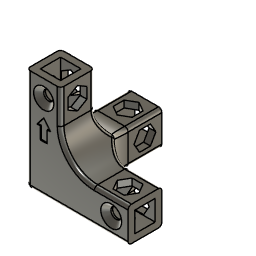
Corner Piece - Cube v1 (Autodesk Fusion 360 design; units mm, degrees)
Autodesk Fusion 360 part; units mm, degrees
sketch "Sketch5" plane through (0, 0, 0) normal (0, 0, 1) x (1, 0, 0)
  line L0 (0, 0) -> (10, 0)
  line L1 (10, 0) -> (10, 10)
  line L2 (0, 10) -> (0, 0)
  line L3 (10, 10) -> (10, 20)
  line L4 (10, 20) -> (0, 20)
  line L5 (0, 20) -> (0, 10)
  line L6 (10, 0) -> (20, 0)
  line L7 (20, 0) -> (20, 10)
  line L8 (20, 10) -> (10, 10)
  line L9 (10, 10) -> (10, 0)
  line L10 (10, 10) -> (0, 10)
  dimension "d18" = 10
  constraint horizontal L0
  constraint vertical L1
  constraint vertical L2
  constraint coincident L0.start L2.end
  constraint equal L0 L2
  constraint vertical L3
  constraint horizontal L4
  constraint vertical L5
  constraint equal L2 L5
  constraint horizontal L6
  constraint vertical L7
  constraint horizontal L8
  constraint vertical L9
  constraint perpendicular L2 L10
  constraint equal L0 L6
  constraint equal L7 L8
  constraint equal L3 L4
  constraint equal L3 L10
  measures "d18" distance of L0.start L0.end
extrude "Extrude8" add sketch "Sketch5" along normal blind 20 contours L0 L1 L2 L9 L10
extrude "Extrude9" add sketch "Sketch5" along normal blind 10 contours L1 L6 L7 L8 L9 | L3 L4 L5 L10
sketch "Sketch6" plane through (20, 0, 0) normal (1, 0, 0) x (0, 1, 0)
  line L0 (0, 0) -> (10, 0)
  line L1 (10, 0) -> (10, 10)
  line L2 (10, 10) -> (0, 10)
  line L3 (0, 10) -> (0, 0)
  line L4 (0, 10) -> (2, 10) construction
  line L5 (2, 10) -> (2, 8) construction
  line L6 (10, 0) -> (8, 0) construction
  line L7 (8, 0) -> (8, 2) construction
  line L8 (2, 8) -> (8, 8)
  line L9 (8, 8) -> (8, 2)
  line L10 (8, 2) -> (2, 2)
  line L11 (2, 2) -> (2, 8)
  dimension "CornerPeg" = 2
  dimension "d24" = 2
  dimension "d25" = 2
  dimension "d26" = 2
  constraint coincident L2.end L3.start
  constraint perpendicular L3 L4
  constraint perpendicular L4 L5
  constraint coincident L0.end L1.start
  constraint coincident L0 L6.end
  constraint perpendicular L6 L7
  constraint horizontal L8
  constraint vertical L9
  constraint horizontal L10
  constraint vertical L11
  measures "CornerPeg" distance of L2.end L4.end
  measures "d24" distance of L4.end L5.end
  measures "d25" distance of L0.end L6.end
  measures "d26" distance of L6.end L7.end
sketch "Sketch7" plane through (0, 20, 0) normal (0, 1, 0) x (-1, 0, 0)
  line L0 (-10, 0) -> (0, 0)
  line L1 (0, 0) -> (0, 10)
  line L2 (0, 10) -> (-10, 10)
  line L3 (-10, 10) -> (-10, 0)
  line L4 (0, 0) -> (-2, 0) construction
  line L5 (-2, 0) -> (-2, 2) construction
  line L6 (-10, 10) -> (-8, 10) construction
  line L7 (-8, 10) -> (-8, 8) construction
  line L8 (-8, 8) -> (-2, 8)
  line L9 (-2, 8) -> (-2, 2)
  line L10 (-2, 2) -> (-8, 2)
  line L11 (-8, 2) -> (-8, 8)
  dimension "d27" = 2
  dimension "d28" = 2
  dimension "d29" = 2
  dimension "d30" = 2
  constraint coincident L0.end L1.start
  constraint perpendicular L1 L4
  constraint perpendicular L4 L5
  constraint coincident L2.end L3.start
  constraint perpendicular L3 L6
  constraint perpendicular L6 L7
  constraint horizontal L8
  constraint vertical L9
  constraint horizontal L10
  constraint vertical L11
  measures "d27" distance of L0.end L4.end
  measures "d28" distance of L4.end L5.end
  measures "d29" distance of L2.end L6.end
  measures "d30" distance of L6.end L7.end
sketch "Sketch8" plane through (0, 0, 20) normal (0, 0, 1) x (-1, 0, 0)
  line L0 (-10, -10) -> (0, -10)
  line L1 (0, -10) -> (0, 0)
  line L2 (0, 0) -> (-10, 0)
  line L3 (-10, 0) -> (-10, -10)
  line L4 (0, -10) -> (-2, -10) construction
  line L5 (-2, -10) -> (-2, -8) construction
  line L6 (-10, 0) -> (-8, 0) construction
  line L7 (-8, 0) -> (-8, -2) construction
  line L8 (-2, -8) -> (-8, -8)
  line L9 (-8, -8) -> (-8, -2)
  line L10 (-8, -2) -> (-2, -2)
  line L11 (-2, -2) -> (-2, -8)
  dimension "d31" = 2
  dimension "d32" = 2
  dimension "d33" = 2
  dimension "d34" = 2
  constraint coincident L0.end L1.start
  constraint perpendicular L1 L4
  constraint perpendicular L0 L5
  constraint coincident L2.end L3.start
  constraint perpendicular L3 L6
  constraint perpendicular L2 L7
  constraint horizontal L8
  constraint vertical L9
  constraint horizontal L10
  constraint vertical L11
  measures "d31" distance of L0.end L4.end
  measures "d32" distance of L4.end L5.end
  measures "d33" distance of L2.end L6.end
  measures "d34" distance of L6.end L7.end
extrude "Extrude10" cut sketch "Sketch8" against normal blind 10 contours L8 L9 L10 L11
extrude "Extrude11" cut sketch "Sketch6" against normal blind 10 contours L8 L9 L10 L11
extrude "Extrude12" cut sketch "Sketch7" against normal blind 10 draft 1 contours L8 L9 L10 L11
extrude "Extrude13" add 1 faces at (20, 4, 9.3333) along direction (1, 0, 0) blind 10
extrude "Extrude14" add 1 faces at (6, 0.6667, 20) along direction (0, 0, 1) blind 10
extrude "Extrude15" add 1 faces at (4, 20, 9.3333) along direction (0, 1, 0) blind 10
fillet "Fillet1" radius 10 1 edges at (10, 10, 5)
fillet "Fillet2" radius 10 1 edges at (10, 5, 10)
fillet "Fillet3" radius 10 1 edges at (10, 10, 10)
sketch "Sketch9" plane through (0, 0, 10) normal (0, 0, 1) x (-1, 0, 0)
  line L0 (-20, -10) -> (-20, 0)
  line L1 (-20, 0) -> (-30, 0)
  line L2 (-30, 0) -> (-30, -10)
  line L3 (-30, -10) -> (-20, -10)
  line L4 (-30, -5) -> (-20, -5) construction
  circle A0 centre (-25, -5) radius 1.5
  dimension "d53" = 3
  constraint midpoint L2 L4.start
  constraint perpendicular L0 L4
  constraint midpoint L4 A0.centre
  constraint midpoint L0 L4.end
  measures "d53" diameter of A0
sketch "Sketch10" plane through (0, 0, 10) normal (0, 0, 1) x (-1, 0, 0)
  line L0 (-10, -20) -> (-10, -30)
  line L1 (-10, -30) -> (0, -30)
  line L2 (0, -30) -> (0, -20)
  line L3 (-5, -30) -> (-5, -20) construction
  circle A0 centre (-5, -25) radius 1.5
  line L4 (0, -20) -> (-10, -20)
  dimension "d54" = 3
  constraint midpoint L1 L3.start
  constraint perpendicular L1 L3
  constraint midpoint L3 A0.centre
  constraint midpoint L3.end L4
  measures "d54" diameter of A0
sketch "Sketch11" plane through (0, 10, 0) normal (0, 1, 0) x (-1, 0, 0)
  line L0 (0, 20) -> (0, 30)
  line L1 (0, 30) -> (-10, 30)
  line L2 (-10, 30) -> (-10, 20)
  line L3 (-5, 30) -> (-5, 20) construction
  circle A0 centre (-5, 25) radius 1.5
  line L4 (-10, 20) -> (0, 20)
  dimension "d55" = 3
  constraint midpoint L1 L3.start
  constraint perpendicular L1 L3
  constraint midpoint L3 A0.centre
  constraint midpoint L3.end L4
  measures "d55" diameter of A0
extrude "Extrude16" cut sketch "Sketch9" sketch "Sketch10" against normal blind 24 contours A0 of sketch 2 contours A0
extrude "Extrude17" cut sketch "Sketch11" against normal blind 43 contours A0
extrude "Extrude18" add 1 faces at (10, 4, 4) along direction (1, 0, 0) blind 5
extrude "Extrude19" add 1 faces at (6.0582, 10, 6.0582) along direction (0, 1, 0) blind 5
fillet "Fillet4" radius 1 3 edges at (0, 15, 0) (0, 0, 15) (15, 0, 0)
fillet "Fillet4" radius 1 15 edges at (25, 10, 0) (12.9289, 12.9289, 0) (10, 25, 0) (10, 25, 10) (10.7612, 16.1732, 10.7612) (16.1732, 10.7612, 10.7612) (25, 10, 10) (10, 0, 25) (12.9289, 0, 12.9289) (25, 0, 10) (10, 10, 25) (10.7612, 10.7612, 16.1732) (0, 25, 10) (0, 12.9289, 12.9289) (0, 10, 25)
extrude "Extrude20" add 1 faces at (6, 4, 10) along direction (0, 0, 1) blind 5
sketch "Sketch12" plane through (0, 10, 0) normal (0, 1, 0) x (-1, 0, 0)
  line L0 (-20, 9) -> (-30, 9)
  line L1 (-30, 9) -> (-30, 1)
  line L2 (-30, 1) -> (-20, 1)
  line L3 (-20, 1) -> (-20, 9)
  line L4 (-30, 5) -> (-20, 5) construction
  circle A0 centre (-25, 5) radius 1.6
  line L5 (-10, 9, 20) -> (-10, 1, 20)
  line L6 (-10, 1, 10) -> (-10, 9, 10)
  line L7 (-10, 5, 20) -> (-10, 5, 10) construction
  circle A1 through (-10, 6.6, 15) (-10, 4.2, 16.3856) (-10, 4.2, 13.6144)
  line L8 (-10, 9, 20) -> (-10, 9, 10)
  line L9 (-10, 9, 10) -> (-10, 1, 10)
  line L10 (-10, 1, 10) -> (-10, 1, 20)
  line L11 (-10, 1, 20) -> (-10, 9, 20)
  line L12 (-10, 30, -9) -> (-10, 30, -1)
  line L13 (-10, 20, -1) -> (-10, 20, -9)
  line L14 (-10, 30, -5) -> (-10, 20, -5) construction
  circle A2 through (-10, 26.6, -5) (-10, 24.2, -3.6144) (-10, 24.2, -6.3856)
  line L15 (-10, 30, -9) -> (-10, 20, -9)
  line L16 (-10, 20, -9) -> (-10, 20, -1)
  line L17 (-10, 20, -1) -> (-10, 30, -1)
  line L18 (-10, 30, -1) -> (-10, 30, -9)
  dimension "d71" = 3.2
  dimension "d72" = 3.2
  dimension "d73" = 3.2
  constraint midpoint L1 L4.start
  constraint midpoint L3 L4.end
  constraint midpoint L4 A0.centre
  measures "d71" diameter of A0
extrude "Extrude21" cut sketch "Sketch12" along normal blind 28 contours A1 | A2 in plane through (10, 10, 0) normal (-1, 0, 0)
extrude "Extrude22" cut sketch "Sketch12" against normal blind 19 contours A0
chamfer "Chamfer2" distance 1.5 angle 45 1 edges at (0, 25.5786, 3.5083)
chamfer "Chamfer2" distance 1.5 angle 45 5 edges at (0, 5.5786, 23.5083) (6.3985, 0, 24.4576) (26.4917, 0, 4.4214) (6.3985, 25.5424, 0) (26.3985, 5.5424, 0)
sketch "Sketch13" plane through (0, 0, 10) normal (0, 0, 1) x (-1, 0, 0)
  line L0 (-1, -30) -> (-1, -20)
  line L1 (-1, -20) -> (-9, -20)
  line L2 (-9, -20) -> (-9, -30)
  line L3 (-9, -30) -> (-1, -30)
  circle A0 centre (-5, -25) radius 1.5
  line L4 (-7.8, -26.6166) -> (-5, -28.2332)
  line L5 (-5, -28.2332) -> (-2.2, -26.6166)
  line L6 (-2.2, -26.6166) -> (-2.2, -23.3834)
  line L7 (-2.2, -23.3834) -> (-5, -21.7668)
  line L8 (-5, -21.7668) -> (-7.8, -23.3834)
  line L9 (-7.8, -23.3834) -> (-7.8, -26.6166)
  line L10 (-23.3834, -7.8) -> (-21.7668, -5)
  line L11 (-21.7668, -5) -> (-23.3834, -2.2)
  line L12 (-23.3834, -2.2) -> (-26.6166, -2.2)
  line L13 (-26.6166, -2.2) -> (-28.2332, -5)
  line L14 (-28.2332, -5) -> (-26.6166, -7.8)
  line L15 (-26.6166, -7.8) -> (-23.3834, -7.8)
  point P0 (-5, -25)
  point P1 (-25, -5)
  point P2 (-25, -5)
  dimension "d80" = 2.8
  dimension "d94" = 2.8
  constraint coincident P0 A0.centre
  constraint coincident P2 P1
  measures "d80" distance of P0 L9
  measures "d94" distance of P2 L15
sketch "Sketch14" plane through (0, 10, 0) normal (0, 1, 0) x (-1, 0, 0)
  circle A0 centre (-25, 5) radius 1.6
  line L0 (-20, 9) -> (-30, 9)
  line L1 (-30, 9) -> (-30, 1)
  line L2 (-30, 1) -> (-20, 1)
  line L3 (-20, 1) -> (-20, 9)
  line L4 (-23.3834, 2.2) -> (-21.7668, 5)
  line L5 (-21.7668, 5) -> (-23.3834, 7.8)
  line L6 (-23.3834, 7.8) -> (-26.6166, 7.8)
  line L7 (-26.6166, 7.8) -> (-28.2332, 5)
  line L8 (-28.2332, 5) -> (-26.6166, 2.2)
  line L9 (-26.6166, 2.2) -> (-23.3834, 2.2)
  line L10 (-7.8, 23.3834) -> (-5, 21.7668)
  line L11 (-5, 21.7668) -> (-2.2, 23.3834)
  line L12 (-2.2, 23.3834) -> (-2.2, 26.6166)
  line L13 (-2.2, 26.6166) -> (-5, 28.2332)
  line L14 (-5, 28.2332) -> (-7.8, 26.6166)
  line L15 (-7.8, 26.6166) -> (-7.8, 23.3834)
  point P0 (-25, 5)
  point P1 (-5, 25)
  dimension "d82" = 2.8
  dimension "d108" = 2.8
  constraint coincident P0 A0.centre
  measures "d82" distance of P0 L9
  measures "d108" distance of P1 L15
sketch "Sketch15" plane through (10, 0, 0) normal (1, 0, 0) x (0, 1, 0)
  circle A0 centre (25, 5) radius 1.6
  line L0 (30, 9) -> (20, 9)
  line L1 (20, 9) -> (20, 1)
  line L2 (20, 1) -> (30, 1)
  line L3 (30, 1) -> (30, 9)
  line L4 (26.6166, 2.2) -> (28.2332, 5)
  line L5 (28.2332, 5) -> (26.6166, 7.8)
  line L6 (26.6166, 7.8) -> (23.3834, 7.8)
  line L7 (23.3834, 7.8) -> (21.7668, 5)
  line L8 (21.7668, 5) -> (23.3834, 2.2)
  line L9 (23.3834, 2.2) -> (26.6166, 2.2)
  line L10 (2.2, 23.3834) -> (5, 21.7668)
  line L11 (5, 21.7668) -> (7.8, 23.3834)
  line L12 (7.8, 23.3834) -> (7.8, 26.6166)
  line L13 (7.8, 26.6166) -> (5, 28.2332)
  line L14 (5, 28.2332) -> (2.2, 26.6166)
  line L15 (2.2, 26.6166) -> (2.2, 23.3834)
  point P0 (25, 5)
  point P1 (25, 5)
  point P2 (25, 5)
  point P3 (5, 25)
  dimension "d93" = 2.8
  dimension "d107" = 2.8
  constraint coincident P2 P0
  constraint coincident P2 P1
  measures "d93" distance of P2 L9
  measures "d107" distance of P3 L15
extrude "Extrude23" cut sketch "Sketch14" against normal blind 2.1 contours L4 L5 L6 L7 L8 L9 | L10 L11 L12 L13 L14 L15
extrude "Extrude24" cut sketch "Sketch15" against normal blind 2.1 contours L4 L5 L6 L7 L8 L9 | L10 L11 L12 L13 L14 L15
extrude "Extrude25" cut sketch "Sketch13" against normal blind 2.1 contours L4 L5 L6 L7 L8 L9 | L10 L11 L12 L13 L14 L15
sketch "Sketch17" plane through (0, 0, 0) normal (0, -1, 0) x (1, 0, 0)
  circle A0 centre (5, 25) radius 3
  line L0 (9, 20) -> (9, 30)
  line L1 (9, 30) -> (1, 30)
  line L2 (1, 30) -> (1, 1)
  line L3 (1, 1) -> (30, 1)
  line L4 (30, 1) -> (30, 9)
  line L5 (30, 9) -> (20, 9)
  arc A1 (9, 20) -> (20, 9) centre (20, 20) ccw
  circle A2 centre (25, 5) radius 3.1
  line L6 (9, 20) -> (1, 20) construction
  line L7 (5, 20) -> (5, 17.5) construction
  line L8 (5, 17.5) -> (3, 17.5)
  line L9 (3, 17.5) -> (5, 20)
  line L10 (5, 17.5) -> (7, 17.5)
  line L11 (7, 17.5) -> (5, 20)
  line L12 (4, 17.5) -> (4, 13.9429)
  line L13 (4, 13.9429) -> (6, 13.9429)
  line L14 (6, 13.9429) -> (6, 17.5)
  constraint coincident L0.start A1.start
  constraint coincident L2 L6.end
  constraint perpendicular L2 L6
  constraint midpoint L6 L7.start
  constraint perpendicular L6 L7
  constraint perpendicular L7 L8
  constraint perpendicular L7 L10
  constraint midpoint L8 L12.start
  constraint perpendicular L8 L12
  constraint perpendicular L7 L13
  constraint midpoint L10 L14.end
  constraint perpendicular L10 L14
extrude "Extrude27" cut sketch "Sketch17" against normal blind 0.3 contours L8 L10 L12 L13 L14 | L8 L9 L10 L11
scale "Scale2" factors (1, 1, 1.0114) about (1, 30, 0) bodies 1
equation "CornerLenght = 10.000 mm"
equation "SideThickness = 10.000 mm"
equation "d18 = CornerLenght"
equation "d19 = 2 * CornerLenght"
equation "d21 = CornerLenght"
equation "d24 = CornerPeg"
equation "d25 = CornerPeg"
equation "d26 = CornerPeg"
equation "d27 = CornerPeg"
equation "d28 = CornerPeg"
equation "d29 = CornerPeg"
equation "d30 = CornerPeg"
equation "d31 = CornerPeg"
equation "d32 = CornerPeg"
equation "d33 = CornerPeg"
equation "d34 = CornerPeg"
equation "d35 = -1 * CornerLenght"
equation "d37 = -1 * CornerLenght"
equation "d39 = -1 * CornerLenght"
equation "d40 = deg"
equation "CornerExtension = 10 mm"
equation "d43 = CornerExtension"
equation "d45 = CornerExtension"
equation "d71 = ScrewHole"
equation "d72 = ScrewHole"
equation "d73 = ScrewHole"
equation "d80 = 2.6 mm + PrintTolerance"
equation "d82 = 2.6 mm + PrintTolerance"
equation "PrintTolerance = 0.2 mm"
equation "d93 = 2.6 mm + PrintTolerance"
equation "d94 = 2.6 mm + PrintTolerance"
equation "ScrewHole = 3.20 mm"
equation "d107 = 2.6 mm + PrintTolerance"
equation "d108 = 2.6 mm + PrintTolerance"
